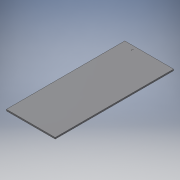
# Autodesk Inventor part: 足裏_メインフレーム_1_3
Saved by Autodesk Inventor 2018 (Build 220112000, 112)
## iProperties
Created: 2016-05-13
Part Number: 足裏_メインフレーム_1_3
Material: GFRP
Document SubType Name: Modeling
Designer: hiroaki
Density: 1.75 g/cm^3
Appearance: 滑らか - 淡い灰色
Mass: 33.025 g
Surface Area: 212.008 cm^2
Volume: 18.8714 cm^3
Author: hiroaki
Autodesk Inventor part; units mm, degrees
ref_plane "YZ Plane" through (0, 0, 0) normal (1, 0, 0) x (0, 1, 0)
ref_plane "XZ Plane" through (0, 0, 0) normal (0, 1, 0) x (-1, 0, 0)
ref_plane "XY Plane" through (0, 0, 0) normal (0, 0, 1) x (1, 0, 0)
sketch "スケッチ1" plane through (0, 0, 0) normal (0, 0, 1) x (1, 0, 0)
  circle A0 centre (-4.75, 48) radius 1.55
  circle A1 centre (4.75, 48) radius 1.55
  circle A2 centre (-4.75, -48) radius 1.55
  circle A3 centre (4.75, -48) radius 1.55
  line L0 (-4.75, -48) -> (4.75, -48) construction
  line L1 (4.75, -48) -> (4.75, 48) construction
  line L2 (4.75, 48) -> (-4.75, 48) construction
  line L3 (-4.75, 48) -> (-4.75, -48) construction
  line L4 (-4.75, -48) -> (4.75, 48) construction
  line L5 (4.75, -48) -> (-4.75, 48) construction
  line L6 (-17.75, 61) -> (50.25, 61)
  line L7 (50.25, 61) -> (50.25, -104)
  line L8 (50.25, -104) -> (-17.75, -104)
  line L9 (-17.75, -104) -> (-17.75, 61)
  circle A4 centre (44.25, 55) radius 1.55
  line L10 (16.25, 61) -> (16.25, -104) construction
  line L11 (16.25, -21.5) -> (50.25, -21.5) construction
  circle A5 centre (21.25, 55) radius 1.55
  circle A6 centre (33.25, 55) radius 1.55
  line L12 (16.25, 19.75) -> (50.25, 19.75) construction
  line L13 (16.25, 40.375) -> (50.25, 40.375) construction
  circle A7 centre (44.25, 25.75) radius 1.55
  circle A8 centre (44.25, -15.5) radius 1.55
  circle A9 centre (44.25, 13.75) radius 1.55
  circle A10 centre (44.25, -98) radius 1.55
  circle A11 centre (21.25, -98) radius 1.55
  circle A12 centre (33.25, -98) radius 1.55
  circle A13 centre (44.25, -68.75) radius 1.55
  circle A14 centre (44.25, -27.5) radius 1.55
  circle A15 centre (44.25, -56.75) radius 1.55
  circle A16 centre (-11.75, 55) radius 1.55
  circle A17 centre (11.25, 55) radius 1.55
  circle A18 centre (-0.75, 55) radius 1.55
  circle A19 centre (-11.75, 25.75) radius 1.55
  circle A20 centre (-11.75, -15.5) radius 1.55
  circle A21 centre (-11.75, 13.75) radius 1.55
  circle A22 centre (-11.75, -27.5) radius 1.55
  circle A23 centre (-11.75, -56.75) radius 1.55
  circle A24 centre (11.25, -98) radius 1.55
  circle A25 centre (-0.75, -98) radius 1.55
  circle A26 centre (-11.75, -98) radius 1.55
  circle A27 centre (-11.75, -68.75) radius 1.55
  circle A28 centre (-4.75, 38) radius 1.55
  circle A29 centre (4.75, 38) radius 1.55
  circle A30 centre (-4.75, -58) radius 1.55
  circle A31 centre (4.75, -58) radius 1.55
  circle A32 centre (-4.75, 28) radius 1.55
  circle A33 centre (4.75, 28) radius 1.55
  circle A34 centre (-4.75, -68) radius 1.55
  circle A35 centre (4.75, -68) radius 1.55
  circle A36 centre (-4.75, 18) radius 1.55
  circle A37 centre (4.75, 18) radius 1.55
  circle A38 centre (-4.75, -78) radius 1.55
  circle A39 centre (4.75, -78) radius 1.55
  circle A40 centre (-4.75, 8) radius 1.55
  circle A41 centre (4.75, 8) radius 1.55
  circle A42 centre (-4.75, -88) radius 1.55
  circle A43 centre (4.75, -88) radius 1.55
  circle A44 centre (25.5, 36.25) radius 10.75
  line L14 (14.75, 47) -> (36.25, 47) construction
  line L15 (36.25, 47) -> (36.25, -90) construction
  line L16 (36.25, -90) -> (14.75, -90) construction
  line L17 (14.75, -90) -> (14.75, 47) construction
  circle A45 centre (25.5, -0.75) radius 10.75
  circle A46 centre (25.5, -37.75) radius 10.75
  circle A47 centre (25.5, -74.75) radius 10.75
  circle A48 centre (4.75, 48) radius 2.75 construction
  point P0 (0, 0)
  dimension "d0" = 3.1
  dimension "d1" = 9.5
  dimension "d2" = 96
  dimension "d3" = 13
  dimension "d4" = 13
  dimension "d7" = 165
  dimension "d8" = 68
  dimension "d16" = 3.1
  dimension "d17" = 6
  dimension "d18" = 6
  dimension "d19" = 5
  dimension "d20" = 17
  dimension "d21" = 41.25
  dimension "d22" = 20.625
  dimension "d25" = 10
  dimension "d30" = 10
  dimension "d31" = 8
  dimension "d32" = 8
  dimension "d35" = 37
  dimension "d40" = 8
  dimension "d41" = 5.5
  constraints: 49 centre point, 36 end point, 21 symmetric about line, 6 midpoint, 6 parallel, 5 equal radius, 4 coincident, 4 horizontal, 4 perpendicular, 4 point on line, 3 tangent, 2 horizontal alignment, 2 vertical, 59 other
  measures "d0" diameter of A1
  measures "d1" distance of L1.end L2.end
  measures "d2" distance of L0.end L1.end
  measures "d3" distance between parallel lines of L2 L6
  measures "d4" distance between parallel lines of L9 L3
  measures "d7" distance of L8.end L6.start
  measures "d8" distance of L6.start L6.end
  measures "d16" diameter of A4
  measures "d17" distance from line of L6 A4.centre
  measures "d18" distance from line of L7 A4.centre
  measures "d19" distance from line of L10 A5.centre
  measures "d20" distance from line of A6.centre L7
  measures "d21" distance between parallel lines of L6 L12
  measures "d22" distance between parallel lines of L6 L13
  measures "d25" distance of L1.end A29.centre
  measures "d30" distance between parallel lines of L1 L17
  measures "d31" distance from line of A5.centre L14
  measures "d32" distance from line of A7.centre L15
  measures "d35" distance of A44.centre A45.centre
  measures "d40" distance from line of L16 A11.centre
  measures "d41" diameter of A48
extrude "押し出し1" add sketch "スケッチ1" along normal blind 2
sketch "スケッチ3" plane through (0, 0, 2) normal (0, 0, 1) x (1, 0, 0)
  circle A0 centre (44.25, 13.75) radius 1.55 projected
  circle A1 centre (44.25, 13.75) radius 1.55
  circle A2 centre (44.25, -15.5) radius 1.55 projected
  circle A3 centre (44.25, -15.5) radius 1.55
  circle A4 centre (44.25, -27.5) radius 1.55 projected
  circle A5 centre (44.25, -27.5) radius 1.55
  circle A6 centre (44.25, 25.75) radius 1.55 projected
  circle A7 centre (44.25, 25.75) radius 1.55
  circle A8 centre (4.75, 28) radius 1.55 projected
  circle A9 centre (4.75, 28) radius 1.55
  circle A10 centre (4.75, 18) radius 1.55 projected
  circle A11 centre (4.75, 18) radius 1.55
  circle A12 centre (4.75, 8) radius 1.55 projected
  circle A13 centre (4.75, 8) radius 1.55
  circle A14 centre (-4.75, 8) radius 1.55 projected
  circle A15 centre (-4.75, 8) radius 1.55
  circle A16 centre (-4.75, 18) radius 1.55 projected
  circle A17 centre (-4.75, 18) radius 1.55
  circle A18 centre (-4.75, 28) radius 1.55 projected
  circle A19 centre (-4.75, 28) radius 1.55
  circle A20 centre (-4.75, 38) radius 1.55 projected
  circle A21 centre (-4.75, 38) radius 1.55
  circle A22 centre (4.75, 38) radius 1.55 projected
  circle A23 centre (4.75, 38) radius 1.55
  circle A24 centre (-11.75, 25.75) radius 1.55 projected
  circle A25 centre (-11.75, 25.75) radius 1.55
  circle A26 centre (-11.75, 13.75) radius 1.55 projected
  circle A27 centre (-11.75, 13.75) radius 1.55
  circle A28 centre (-11.75, 55) radius 1.55 projected
  circle A29 centre (-11.75, 55) radius 1.55
  circle A30 centre (-0.742, 55) radius 1.5522
  circle A31 centre (11.25, 55) radius 1.55 projected
  circle A32 centre (11.25, 55) radius 1.55
  circle A33 centre (21.25, 55) radius 1.55 projected
  circle A34 centre (21.25, 55) radius 1.55
  circle A35 centre (33.25, 55) radius 1.55 projected
  circle A36 centre (33.25, 55) radius 1.55
  circle A37 centre (44.25, 55) radius 1.55 projected
  circle A38 centre (44.25, 55) radius 1.55
  circle A39 centre (25.5, 36.25) radius 10.75 projected
  circle A40 centre (25.5, 36.25) radius 10.75
  circle A41 centre (25.5, -0.75) radius 10.75 projected
  circle A42 centre (25.5, -0.75) radius 10.75
  circle A43 centre (25.5, -37.75) radius 10.75 projected
  circle A44 centre (25.5, -37.75) radius 10.75
  circle A45 centre (44.25, -56.75) radius 1.55 projected
  circle A46 centre (44.25, -56.75) radius 1.55
  circle A47 centre (44.25, -68.75) radius 1.55 projected
  circle A48 centre (44.25, -68.75) radius 1.55
  circle A49 centre (25.5, -74.75) radius 10.75 projected
  circle A50 centre (25.5, -74.75) radius 10.75
  circle A51 centre (4.75, -78) radius 1.55 projected
  circle A52 centre (4.75, -78) radius 1.55
  circle A53 centre (4.75, -68) radius 1.55 projected
  circle A54 centre (4.75, -68) radius 1.55
  circle A55 centre (4.75, -58) radius 1.55 projected
  circle A56 centre (4.75, -58) radius 1.55
  circle A57 centre (4.75, -48) radius 1.55 projected
  circle A58 centre (4.75, -48) radius 1.55
  circle A59 centre (-4.75, -48) radius 1.55 projected
  circle A60 centre (-4.75, -48) radius 1.55
  circle A61 centre (-4.75, -58) radius 1.55 projected
  circle A62 centre (-4.75, -58) radius 1.55
  circle A63 centre (-11.75, -56.75) radius 1.55 projected
  circle A64 centre (-11.75, -56.75) radius 1.55
  circle A65 centre (-4.75, -68) radius 1.55 projected
  circle A66 centre (-4.75, -68) radius 1.55
  circle A67 centre (-11.75, -68.75) radius 1.55 projected
  circle A68 centre (-11.75, -68.75) radius 1.55
  circle A69 centre (-4.75, -78) radius 1.55 projected
  circle A70 centre (-4.75, -78) radius 1.55
  circle A71 centre (-4.75, -88) radius 1.55 projected
  circle A72 centre (-4.75, -88) radius 1.55
  circle A73 centre (4.75, -88) radius 1.55 projected
  circle A74 centre (4.75, -88) radius 1.55
  circle A75 centre (-11.75, -98) radius 1.55 projected
  circle A76 centre (-11.75, -98) radius 1.55
  circle A77 centre (-0.75, -98) radius 1.55 projected
  circle A78 centre (-0.75, -98) radius 1.55
  circle A79 centre (11.25, -98) radius 1.55 projected
  circle A80 centre (11.25, -98) radius 1.55
  circle A81 centre (21.25, -98) radius 1.55 projected
  circle A82 centre (21.25, -98) radius 1.55
  circle A83 centre (44.25, -98) radius 1.55 projected
  circle A84 centre (44.25, -98) radius 1.55
  circle A85 centre (33.25, -98) radius 1.55 projected
  circle A86 centre (33.25, -98) radius 1.55
  circle A87 centre (-4.75, 48) radius 1.55 projected
  circle A88 centre (-4.75, 48) radius 1.55
  circle A89 centre (4.75, 48) radius 1.55 projected
  circle A90 centre (4.75, 48) radius 1.55
  circle A91 centre (-11.75, -27.5) radius 1.55 projected
  circle A92 centre (-11.75, -27.5) radius 1.55
  circle A93 centre (-11.75, -15.5) radius 1.55 projected
  circle A94 centre (-11.75, -15.5) radius 1.55
  point P0 (0, 0)
  constraints: 48 centre point, 47 coincident
extrude "押し出し3" add sketch "スケッチ3" against normal up to surface (2 mm away)
equation "\"d1\" = d20_1"
equation "\"d4\" = d3"
equation "\"d8\" = 足_短辺"
equation "\"d18\" = d17"
equation "\"d20\" = 0.25 * d8"
equation "\"d21\" = 0.25 * d7"
equation "\"d22\" = 0.5 * d21"
equation "\"d31\" = d32"
equation "\"d40\" = d31"
equation "\"H_head\" = 96"
equation "\"H_leg\" = 306"
equation "\"足の面積\" = 12720.125"
equation "\"現在の面積\" = 11560"
equation "\"足_短辺\" = 68"
equation "\"円柱\" = 313.5"
equation "\"胴体中心から手先\" = 342"
equation "\"H_leg_1\" = 186.2"
equation "\"H_leg_MAX\" = 399"
equation "\"H_head_1\" = 26.6"
equation "\"H_head_MAX\" = 142.5"
equation "\"d20_1\" = 9.5"
